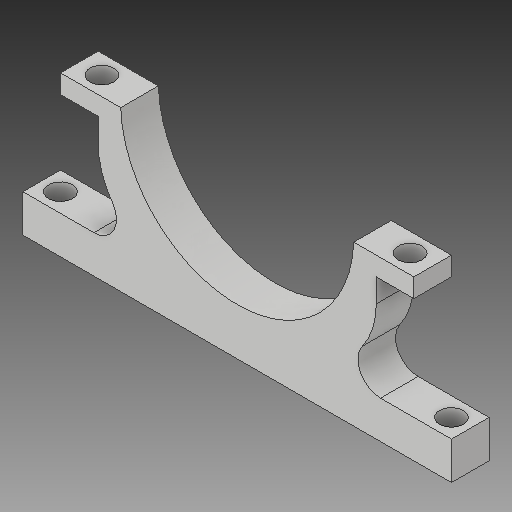
# Autodesk Inventor part: MOTOR MOUNT REAL BOTTOM
Saved by Autodesk Inventor 2019 (Build 230136000, 136)
## iProperties
Created: 2018-01-16
Part Number: MOTOR MOUNT REAL BOTTOM
Material: Generic
Document SubType Name: Modeling
Designer: Administrator
Density: 1 g/cm^3
Appearance: Default
Author: Administrator
Autodesk Inventor part; units mm, degrees
ref_plane "YZ Plane" through (0, 0, 0) normal (1, 0, 0) x (0, 1, 0)
ref_plane "XZ Plane" through (0, 0, 0) normal (0, 1, 0) x (-1, 0, 0)
ref_plane "XY Plane" through (0, 0, 0) normal (0, 0, 1) x (1, 0, 0)
sketch "Sketch1" plane through (0, 0, 0) normal (0, 0, 1) x (1, 0, 0)
  arc A0 (-39.344, -1.4316) -> (39.344, -1.4316) centre (0, 0) ccw
  line L0 (-39.344, -1.4316) -> (-39.3671, -1.4316)
  line L1 (-39.344, -1.4316) -> (-52.044, -1.4316)
  line L2 (39.344, -1.4316) -> (52.044, -1.4316)
  arc A1 (-46.964, -22.4724) -> (46.964, -22.4724) centre (0, 0) ccw
  line L3 (0, -52.0636) -> (0, -55.2386)
  line L4 (0, -55.2386) -> (-72.364, -55.2386)
  line L5 (0, -55.2386) -> (72.364, -55.2386)
  line L6 (-52.044, -1.4316) -> (-59.664, -1.4316)
  line L7 (52.044, -1.4316) -> (59.664, -1.4316)
  line L8 (39.344, -1.4316) -> (46.964, -1.4316)
  line L9 (46.964, -1.4316) -> (46.964, -22.4724)
  line L10 (-39.344, -1.4316) -> (-45.694, -1.4316)
  line L11 (-39.344, -1.4316) -> (-46.964, -1.4316)
  line L12 (-46.964, -1.4316) -> (-46.964, -22.4724)
  line L13 (-46.964, -7.7816) -> (-59.664, -7.7816)
  line L14 (-59.664, -7.7816) -> (-59.664, -1.4316)
  line L15 (46.964, -7.7816) -> (59.664, -7.7816)
  line L16 (59.664, -7.7816) -> (59.664, -1.4316)
  line L17 (-72.364, -55.2386) -> (-72.364, -42.5386)
  line L18 (72.364, -55.2386) -> (72.364, -42.5386)
  line L19 (-72.364, -42.5386) -> (-30.0181, -42.5386)
  line L20 (72.364, -42.5386) -> (30.0181, -42.5386)
  dimension "d0" = 78.74
  dimension "d2" = 12.7
  dimension "d3" = 12.7
  dimension "d4" = 3.175
  dimension "d5" = 7.62
  dimension "d6" = 7.62
  dimension "d7" = 7.62
  dimension "d9" = 7.62
  dimension "d10" = 6.35
  dimension "d11" = 6.35
  dimension "d14" = 12.7
  dimension "d15" = 12.7
  constraints: 42 end point, 8 horizontal, 7 point on circle, 6 point on line, 5 vertical, 2 centre point, 2 perpendicular, 1 coincident, 1 concentric, 1 midpoint
  measures "d0" diameter of A0
  measures "d2" distance of L2.start L2.end
  measures "d3" distance of L0.start L1.end
  measures "d4" distance of L3.start L3.end
  measures "d5" distance of L1.end L6.end
  measures "d6" distance of L2.end L7.end
  measures "d7" distance of L2.start L8.end
  measures "d9" distance of L0.start L11.end
  measures "d10" distance of L13.end L6.end
  measures "d11" distance of L15.end L7.end
  measures "d14" distance of L5.end L18.end
  measures "d15" distance of L4.end L17.end
extrude "Extrusion1" add sketch "Sketch1" along normal blind 12.7
fillet "Fillet1" radius 7.62 2 edges at (30.0181, -42.5386, 6.35) (-30.0181, -42.5386, 6.35)
fillet "Fillet2" radius 25.4 2 edges at (-46.964, -22.4724, 6.35) (46.964, -22.4724, 6.35)
sketch "Sketch2" plane through (-59.664, -1.4316, 0) normal (0, 1, 0) x (1, 0, 0)
  line L0 (0, 0) -> (0, -12.7) projected
  line L1 (99.0079, 0) -> (20.32, 0) projected
  line L2 (0, 0) -> (20.32, 0)
  circle A0 centre (7.62, -6.35) radius 4.064
  circle A1 centre (111.7079, -6.35) radius 4.064
  line L3 (119.3279, 0) -> (119.3279, -12.7) projected
  line L4 (-12.7, 0) -> (132.0279, 0) projected
  line L5 (119.3279, 0) -> (132.0279, 0)
  circle A2 centre (125.6779, -6.35) radius 4.064
  line L6 (-12.7, 0) -> (0, 0)
  circle A3 centre (-6.35, -6.35) radius 4.064
  line L7 (20.32, 0) -> (20.32, -12.7) projected
  line L8 (99.0079, 0) -> (99.0079, -12.7) projected
  point P0 (59.664, 0)
  dimension "d20" = 8.128
  dimension "d21" = 8.128
  dimension "d22" = 8.128
  dimension "d23" = 8.128
  dimension "d24" = 12.7
  dimension "d25" = 12.7
  constraints: 6 end point, 4 centre point, 2 collinear, 1 horizontal
  measures "d20" diameter of A0
  measures "d21" diameter of A1
  measures "d22" diameter of A2
  measures "d23" diameter of A3
  measures "d24" distance from line of L7 A0.centre
  measures "d25" distance from line of L8 A1.centre
extrude "Extrusion2" cut sketch "Sketch2" against normal blind 25.4 contours A0 | A1
extrude "Extrusion3" cut sketch "Sketch2" against normal blind 76.2 contours A2 | A3
body "Solid1"
